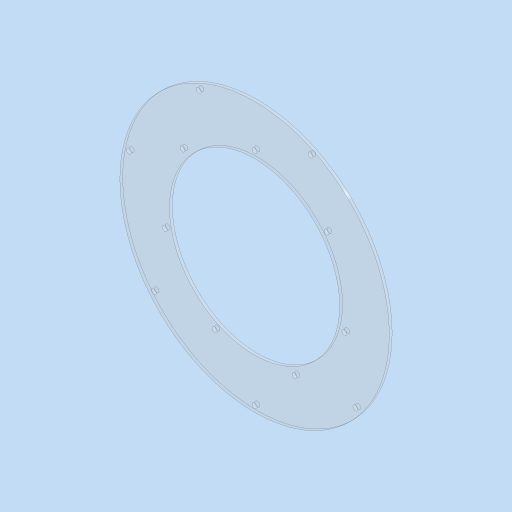
# Autodesk Inventor part: Lid_Loose
Saved by Autodesk Inventor 2024.2 (Build 282272000, 272)
## iProperties
Created: 2025-04-30
Part Number: Lid_Loose
Material: Generic
Document SubType Name: Modeling
Designer: 23661194
Density: 1 g/cm^3
Appearance: Polycarbonate - Clear
Author: 23661194
Autodesk Inventor part; units mm, degrees
ref_plane "YZ Plane" through (0, 0, 0) normal (1, 0, 0) x (0, 1, 0)
ref_plane "XZ Plane" through (0, 0, 0) normal (0, 1, 0) x (-1, 0, 0)
ref_plane "XY Plane" through (0, 0, 0) normal (0, 0, 1) x (1, 0, 0)
sketch "Sketch1" plane through (0, 0, 0) normal (0, 0, 1) x (1, 0, 0)
  circle A0 centre (0, 0) radius 60
  circle A1 centre (0, 0) radius 95
  circle A2 centre (0, 0) radius 65
  circle A3 centre (0, 0) radius 91
  circle A4 centre (0, 65) radius 1.75
  circle A5 centre (-50.819, 40.5268) radius 1.75
  circle A6 centre (-63.3703, -14.4639) radius 1.75
  circle A7 centre (-28.2024, -58.563) radius 1.75
  circle A8 centre (28.2024, -58.563) radius 1.75
  circle A9 centre (63.3703, -14.4639) radius 1.75
  line L0 (0, 0) -> (39.4834, 81.9882)
  line L1 (0, 133) -> (0, -133) projected
  circle A10 centre (39.4834, 81.9882) radius 1.75
  circle A11 centre (-39.4834, 81.9882) radius 1.75
  circle A12 centre (-88.7184, 20.2494) radius 1.75
  circle A13 centre (-71.1467, -56.7376) radius 1.75
  circle A14 centre (0, -91) radius 1.75
  circle A15 centre (71.1467, -56.7376) radius 1.75
  circle A16 centre (88.7184, 20.2494) radius 1.75
  circle A17 centre (50.819, 40.5268) radius 1.75
  dimension "d2" = 130
  dimension "d3" = 182
  dimension "d0" = 120
  dimension "d1" = 190
  dimension "d4" = 3.5
  dimension "d7" = 360
  dimension "d9" = 25.714
  dimension "d10" = 3.5
  dimension "d13" = 360
  constraints: 16 centre point, 11 coincident, 2 end point, 1 vertical alignment, 35 other
  measures "d0" diameter of A0
  measures "d1" diameter of A1
  measures "d4" diameter of A4
  measures "d9" angle of L1 L0
  measures "d10" diameter of A10
extrude "Extrusion1" add sketch "Sketch1" along normal blind 2 contours A0 L0 A2 A17 A9 A8 L1 | A0 L1 A4 A2 L0 | L1 A2 A7 A6 A5 A4 A0 | L0 A10 A3 A16 A15 A14 L1 A2 A8 A9 A17 | A2 A4 L1 A3 A10 L0 | L1 A14 A3 A13 A12 A11 A4 A2 A5 A6 A7 | A17 A2 | A2 A17 | A3 L1 A1 A14 A15 A16 A10 | A14 L1 A1 A3 A11 A12 A13 | A16 A3 | A3 A16
extrude "Extrusion2" cut sketch "Sketch1" along normal through all contours A17 A2 | A2 A17
body "Solid1"
